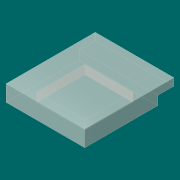
# Autodesk Inventor part: mppcLens
Saved by Autodesk Inventor 2016 (Build 200138000, 138)
## iProperties
Created: 2015-10-16
Part Number: mppcLens
Material: Glass
Document SubType Name: Modeling
Designer: Sawaiz
Density: 2.18 g/cm^3
Appearance: Clear
Author: Sawaiz
Autodesk Inventor part; units mm, degrees
ref_plane "YZ Plane" through (0, 0, 0) normal (1, 0, 0) x (0, 1, 0)
ref_plane "XZ Plane" through (0, 0, 0) normal (0, 1, 0) x (-1, 0, 0)
sketch "Sketch1" plane through (0, 0, 0) normal (0, 0, 1) x (1, 0, 0)
  line L0 (-1.775, 2.45) -> (-1.775, -2.45) projected
  line L1 (2.775, -2.45) -> (-1.775, -2.45) projected
  line L2 (2.775, 2.45) -> (2.775, -2.45) projected
  line L3 (-1.775, 2.45) -> (2.775, 2.45) projected
  line L4 (1.83, 1.5) -> (1.83, -1.5) projected
  line L5 (1.83, -1.5) -> (-1.17, -1.5) projected
  line L6 (-1.17, -1.5) -> (-1.17, 1.5) projected
  line L7 (-1.17, 1.5) -> (1.83, 1.5) projected
  point P0 (0, 0)
extrude "Extrusion1" add sketch "Sketch1" against normal blind 1
sketch "Sketch2" plane through (0, 0, 0) normal (0, 0, 1) x (1, 0, 0)
  line L0 (1.83, 1.5) -> (-1.17, 1.5) projected
  line L1 (-1.17, 1.5) -> (-1.17, -1.5) projected
  line L2 (-1.17, -1.5) -> (1.83, -1.5) projected
  line L3 (1.83, -1.5) -> (1.83, 1.5) projected
  point P0 (0, 0)
extrude "Extrusion2" add sketch "Sketch2" against normal blind 0.45
ref_plane "Work Plane1" through (-2.275, 0, -0.45) normal (0, 0, 1) x (1, 0, 0)
sketch "Sketch3" plane through (-2.275, 0, -0.45) normal (0, 0, 1) x (1, 0, 0)
  line L0 (-0.5, 2.45) -> (0.5, 2.45) projected
  line L1 (-0.5, -2.45) -> (-0.5, 2.45) projected
  line L2 (0.5, -2.45) -> (-0.5, -2.45) projected
  line L3 (0.5, -2.45) -> (0.5, 2.45) projected
  point P0 (2.275, 0)
extrude "Extrusion3" add sketch "Sketch3" along normal blind 0.45
body "Solid1"
